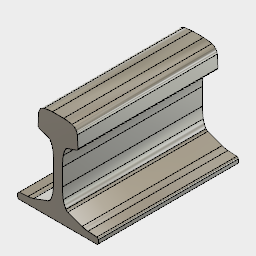
F3Z - Traverse (Autodesk Fusion 360 archive; units mm, degrees)
design "F3D - Rail 60E1"
Autodesk Fusion 360 part; units mm, degrees
sketch "Sketch1" plane through (0, 0, 0) normal (0, 0, 1) x (1, 0, 0)
  line L0 (-73, 0) -> (73, 0)
  arc A0 (73, 0) -> (75, 2) centre (73, 2) ccw
  line L1 (75, 2) -> (75, 8.7069)
  arc A1 (75, 8.7069) -> (72.214, 11.6992) centre (72, 8.7069) ccw
  line L2 (72.214, 11.6992) -> (55.6834, 12.8812)
  arc A2 (44.8686, 15.1869) -> (55.6834, 12.8812) centre (58.5363, 52.7794) ccw
  line L3 (44.8686, 15.1869) -> (18.3683, 24.8217)
  arc A3 (14.8553, 27.6412) -> (18.3683, 24.8217) centre (20.7602, 31.4004) ccw
  arc A4 (9.845, 40.75) -> (14.8553, 27.6412) centre (44.3798, 46.4375) ccw
  arc A5 (8.25, 60.25) -> (9.845, 40.75) centre (128.25, 60.25) ccw
  line L4 (8.25, 60.25) -> (8.25, 92.25)
  arc A6 (9.845, 111.75) -> (8.25, 92.25) centre (128.25, 92.25) ccw
  arc A7 (14.3127, 123.9781) -> (9.845, 111.75) centre (44.3798, 106.0625) ccw
  arc A8 (18.1131, 127.0359) -> (14.3127, 123.9781) centre (20.3261, 120.395) ccw
  line L5 (18.1131, 127.0359) -> (35.063, 132.6843)
  arc A9 (35.063, 132.6843) -> (37.1108, 135.6801) centre (34.1145, 135.5304) ccw
  line L6 (37.1108, 135.6801) -> (36, 157.9144)
  arc A10 (36, 157.9144) -> (26, 169.744) centre (23.0263, 157.0887) ccw
  arc A11 (26, 169.744) -> (10.5, 171.8162) centre (7.7, 91.8652) ccw
  arc A12 (10.5, 171.8162) -> (-10.5, 171.8162) centre (0, -128) ccw
  arc A13 (-10.5, 171.8162) -> (-26, 169.744) centre (-7.7, 91.8652) ccw
  arc A14 (-26, 169.744) -> (-36, 157.9144) centre (-23.0263, 157.0887) ccw
  line L7 (-36, 157.9144) -> (-37.1108, 135.6801)
  arc A15 (-37.1108, 135.6801) -> (-35.063, 132.6843) centre (-34.1145, 135.5304) ccw
  line L8 (-35.063, 132.6843) -> (-18.1131, 127.0359)
  arc A16 (-14.3127, 123.9781) -> (-18.1131, 127.0359) centre (-20.3261, 120.395) ccw
  arc A17 (-9.845, 111.75) -> (-14.3127, 123.9781) centre (-44.3798, 106.0625) ccw
  arc A18 (-8.25, 92.25) -> (-9.845, 111.75) centre (-128.25, 92.25) ccw
  line L9 (-8.25, 92.25) -> (-8.25, 60.25)
  arc A19 (-9.845, 40.75) -> (-8.25, 60.25) centre (-128.25, 60.25) ccw
  arc A20 (-14.8553, 27.6412) -> (-9.845, 40.75) centre (-44.3798, 46.4375) ccw
  arc A21 (-18.3683, 24.8217) -> (-14.8553, 27.6412) centre (-20.7602, 31.4004) ccw
  line L10 (-18.3683, 24.8217) -> (-44.8686, 15.1869)
  arc A22 (-55.6834, 12.8812) -> (-44.8686, 15.1869) centre (-58.5363, 52.7794) ccw
  line L11 (-55.6834, 12.8812) -> (-72.214, 11.6992)
  arc A23 (-72.214, 11.6992) -> (-75, 8.7069) centre (-72, 8.7069) ccw
  line L12 (-75, 8.7069) -> (-75, 2)
  arc A24 (-75, 2) -> (-73, 0) centre (-73, 2) ccw
extrude "Extrude1" add sketch "Sketch1" along normal mid plane 260
